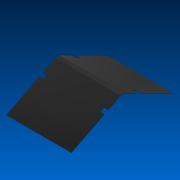
# Autodesk Inventor part: Ramp Using 1__16 Gray Tinted Polycarbonate Sheet (36 x 72) (217-6627)
Saved by Autodesk Inventor 2022.2 (Build 262287000, 287)
## iProperties
Created: 2022-01-06
Part Number: Ramp Using 1__16 Gray Tinted Polycarbonate Sheet (36 x 72) (217-6627)
Material: Polycarbonate, Clear
Document SubType Name: Modeling
Designer: omard
Density: 1.2 g/cm^3
Appearance: Smooth - Black
Author: omard
Autodesk Inventor part; units mm, degrees
ref_plane "YZ Plane" through (0, 0, 0) normal (1, 0, 0) x (0, 1, 0)
ref_plane "XZ Plane" through (0, 0, 0) normal (0, 1, 0) x (-1, 0, 0)
ref_plane "XY Plane" through (0, 0, 0) normal (0, 0, 1) x (1, 0, 0)
sketch "Sketch1" plane through (0, 0, 0) normal (0, 1, 0) x (-1, 0, 0)
  line L0 (203.2, 12.7) -> (-203.2, 12.7)
  line L1 (-203.2, 12.7) -> (-203.2, -12.7)
  line L2 (-203.2, -12.7) -> (203.2, -12.7)
  line L3 (203.2, -12.7) -> (203.2, 12.7)
  line L4 (203.2, 12.7) -> (-203.2, -12.7) construction
  line L5 (-203.2, 12.7) -> (203.2, -12.7) construction
  point P0 (0, 0)
  dimension "d0" = 406.4
  dimension "d1" = 25.4
  constraints: 12 end point, 2 midpoint, 2 parallel, 1 horizontal, 1 perpendicular
  measures "d0" distance of L2.end L1.end
  measures "d1" distance of L1.end L0.end
extrude "Extrusion1" add sketch "Sketch1" along normal blind 1.5875
sketch "Sketch2" plane through (0, 1.5875, 0) normal (0, 1, 0) x (1, 0, 0)
  line L0 (-203.2, 12.7) -> (-203.2, -12.7) projected
  line L1 (203.2, -12.7) -> (203.2, 12.7) projected
  point P0 (0, 0)
  point P1 (-177.8, 0)
  point P2 (-152.4, 0)
  point P3 (177.8, 0)
  point P4 (152.4, 0)
  point P5 (76.2, 0)
  point P6 (50.8, 0)
  point P7 (-76.2, 0)
  point P8 (-50.8, 0)
  dimension "d4" = 25.4
  dimension "d5" = 25.4
  dimension "d6" = 25.4
  dimension "d7" = 25.4
  dimension "d8" = 25.4
  dimension "d9" = 25.4
  dimension "d10" = 76.2
  dimension "d11" = 76.2
  constraints: 8 horizontal alignment
  measures "d4" distance of point (-152.4, 0) point (-177.8, 0)
  measures "d5" distance of point (177.8, 0) point (152.4, 0)
  measures "d6" distance of point (-50.8, 0) point (-76.2, 0)
  measures "d7" distance of point (50.8, 0) point (76.2, 0)
  measures "d8" distance from line of point (-177.8, 0) L0
  measures "d9" distance from line of L1 point (177.8, 0)
  measures "d10" distance of point (76.2, 0) point (152.4, 0)
  measures "d11" distance of point (-152.4, 0) point (-76.2, 0)
hole "Hole1" at (-177.8, 1.5875, 0) at (177.8, 1.5875, 0) at (76.2, 1.5875, 0) at (-76.2, 1.5875, 0) direction (0, -1, 0) diameter 4.318 end through all start extended yes
sketch "Sketch3" plane through (203.2, 0, 12.7) normal (1, 0, 0) x (0, 0, -1)
  line L0 (0, 0) -> (25.4, 0) projected
  line L1 (0, 0) -> (-0.7189, 1.4154)
  line L2 (-0.7189, 1.4154) -> (-307.7868, -154.5406)
  line L3 (-307.7868, -154.5406) -> (-307.068, -155.956)
  line L4 (-307.068, -155.956) -> (0, 0)
  line L5 (25.4, 0) -> (26.1189, 1.4154)
  line L6 (26.1189, 1.4154) -> (333.1868, -154.5406)
  line L7 (333.1868, -154.5406) -> (332.468, -155.956)
  line L8 (332.468, -155.956) -> (25.4, 0)
  line L9 (0, 0) -> (0, 1.5875) projected
  line L10 (25.4, 0) -> (25.4, 1.5875) projected
  line L11 (0, 1.5875) -> (25.4, 1.5875) projected
  arc A0 (0, 1.5875) -> (-0.7189, 1.4154) centre (0, 0) ccw
  arc A1 (26.1189, 1.4154) -> (25.4, 1.5875) centre (25.4, 0) ccw
  line L12 (-204.5453, -103.886) -> (-179.1453, -103.886)
  line L13 (-357.0791, -181.356) -> (382.4791, -181.356)
  point P0 (12.7, 0)
  point P1 (12.7, -181.356)
  point P2 (12.7, 0)
  dimension "d19" = 25.4
  dimension "d20" = 103.886
  dimension "d21" = 207.0877
  dimension "d22" = 181.356
  dimension "d23" = 25.4
  constraints: 20 end point, 4 parallel, 4 point on circle, 3 equal length, 2 centre point, 2 coincident, 2 horizontal, 2 midpoint, 2 perpendicular, 2 point on line, 1 horizontal alignment, 1 vertical alignment
  measures "d19" distance of L12.start L12.end
  measures "d20" distance between parallel lines of L0 L12
  measures "d21" distance of L12.end L0.start
  measures "d22" distance between parallel lines of L13 L0
  measures "d23" distance from line of L13 L3.end
extrude "Extrusion2" add sketch "Sketch3" against normal up to surface (406.4 mm away) contours L4 L3 L2 L1 | L1 A0 L9 | L10 A1 L5 | L5 L6 L7 L8
sketch "Sketch4" plane through (0, 1.5875, 0) normal (0, 1, 0) x (1, 0, 0)
  line L0 (203.2, -319.768) -> (203.2, -12.7) projected
  line L1 (203.2, -88.9) -> (177.8, -88.9)
  line L2 (177.8, -88.9) -> (177.8, -114.3)
  line L3 (177.8, -114.3) -> (203.2, -114.3)
  line L4 (203.2, -114.3) -> (203.2, -88.9)
  line L5 (203.2, 12.7) -> (203.2, 319.768) projected
  line L6 (203.2, 88.9) -> (177.8, 88.9)
  line L7 (177.8, 88.9) -> (177.8, 114.3)
  line L8 (177.8, 114.3) -> (203.2, 114.3)
  line L9 (203.2, 114.3) -> (203.2, 88.9)
  line L10 (-203.2, 12.7) -> (-203.2, 319.768) projected
  line L11 (-203.2, 114.3) -> (-177.8, 114.3)
  line L12 (-177.8, 114.3) -> (-177.8, 88.9)
  line L13 (-177.8, 88.9) -> (-203.2, 88.9)
  line L14 (-203.2, 88.9) -> (-203.2, 114.3)
  line L15 (-203.2, -319.768) -> (-203.2, -12.7) projected
  line L16 (-203.2, -88.9) -> (-177.8, -88.9)
  line L17 (-177.8, -88.9) -> (-177.8, -114.3)
  line L18 (-177.8, -114.3) -> (-203.2, -114.3)
  line L19 (-203.2, -114.3) -> (-203.2, -88.9)
  line L20 (177.8, -88.9) -> (177.8, 88.9) construction
  line L21 (-177.8, 88.9) -> (-177.8, -88.9) construction
  point P0 (0, 0)
  point P1 (-177.8, 0)
  point P2 (177.8, 0)
  point P3 (177.8, -101.6)
  dimension "d26" = 25.4
  dimension "d29" = 101.6
  constraints: 36 end point, 8 parallel, 6 equal length, 5 point on line, 4 horizontal, 4 perpendicular, 3 midpoint, 2 collinear, 2 horizontal alignment, 1 vertical
  measures "d26" distance of L1.end L2.end
  measures "d29" distance of point (177.8, -101.6) point (177.8, 0)
extrude "Extrusion3" cut sketch "Sketch4" against normal through all
body "Solid1"
